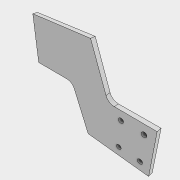
# Autodesk Inventor part: 884702-01
Saved by Autodesk Inventor 2020.1 (Build 241239000, 239)
## iProperties
Created: 2019-09-15
Part Number: 884702-01
Material: Generic
Document SubType Name: Modeling
Designer: thomastremblay
Density: 1 g/cm^3
Appearance: Default
Author: thomastremblay
Autodesk Inventor part; units mm, degrees
ref_plane "YZ Plane" through (0, 0, 0) normal (1, 0, 0) x (0, 1, 0)
ref_plane "XZ Plane" through (0, 0, 0) normal (0, 1, 0) x (-1, 0, 0)
ref_plane "XY Plane" through (0, 0, 0) normal (0, 0, 1) x (1, 0, 0)
sketch "Sketch1" plane through (0, 0, 0) normal (0, 0, 1) x (1, 0, 0)
  line L0 (-177.8, 0) -> (0, 0)
  line L1 (0, 0) -> (0, 127)
  line L2 (-169.9735, 254) -> (-355.6, 254)
  line L3 (-355.6, 254) -> (-355.6, 127)
  line L4 (-355.6, 127) -> (-228.6, 127)
  line L5 (-228.6, 127) -> (-177.8, 0)
  line L6 (-169.9735, 254) -> (-119.1735, 127)
  line L7 (-119.1735, 127) -> (0, 127)
  dimension "d8" = 127
  dimension "brkt_ht" = 254
  dimension "brkt_width" = 355.6
  dimension "d11" = 127
  dimension "d12" = 101.6
  dimension "d13" = 111.801
  dimension "d15" = 177.8
  constraints: 16 end point, 3 parallel, 3 perpendicular, 2 horizontal, 1 coincident
  measures "d8" distance of L2.end L3.end
  measures "brkt_ht" distance between parallel lines of L2 L0
  measures "brkt_width" distance between parallel lines of L1 L3
  measures "d11" distance of L0.end L1.end
  measures "d12" distance between parallel lines of L6 L5
  measures "d13" angle of L5 L4
  measures "d15" distance of point (0, 0) L0.start
extrude "Extrusion1" add sketch "Sketch1" along normal blind 12.7
fillet "Fillet1" radius 25.4 2 edges at (-228.6, 127, 6.35) (-119.1735, 127, 6.35)
sketch "Sketch4" plane through (0, 0, 12.7) normal (0, 0, 1) x (1, 0, 0)
  line L0 (-25.4, 101.6) -> (-82.55, 101.6) construction
  line L1 (-82.55, 101.6) -> (-82.55, 25.4) construction
  line L2 (-82.55, 25.4) -> (-25.4, 25.4) construction
  line L3 (-25.4, 25.4) -> (-25.4, 101.6) construction
  line L4 (0, 0) -> (0, 127) construction
  line L5 (0, 127) -> (-101.9768, 127) construction
  point P0 (-25.4, 63.5)
  point P1 (0, 63.5)
  dimension "d19" = 25.4
  dimension "d20" = 25.4
  dimension "d21" = 57.15
  constraints: 8 end point, 2 midpoint, 2 parallel, 1 horizontal, 1 horizontal alignment, 1 perpendicular
  measures "d19" distance between parallel lines of L5 L0
  measures "d20" distance between parallel lines of L4 L3
  measures "d21" distance of L1.end L2.end
hole "Hole1" at (-25.4, 101.6, 12.7) at (-82.55, 101.6, 12.7) at (-82.55, 25.4, 12.7) at (-25.4, 25.4, 12.7) direction (0, 0, -1) diameter 13.4874 end through all clearance for "Hex Head Bolt" size "1/2" standard "Ansi Unified Screw Threads"
equation "\"d15\" = 0.5 * brkt_width"
body "Solid1"
